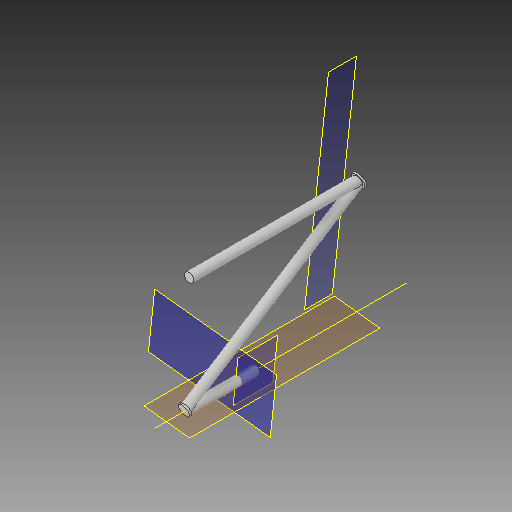
# Autodesk Inventor part: cellSTORM_lightpath
Saved by Autodesk Inventor 2019 (Build 230136000, 136)
## iProperties
Created: 2020-04-25
Part Number: cellSTORM_lightpath
Material: Generic
Document SubType Name: Modeling
Designer: diederichbenedict
Density: 1 g/cm^3
Appearance: Default
Author: diederichbenedict
Autodesk Inventor part; units mm, degrees
ref_plane "YZ Plane" through (0, 0, 0) normal (1, 0, 0) x (0, 1, 0)
ref_plane "XZ Plane" through (0, 0, 0) normal (0, 1, 0) x (-1, 0, 0)
ref_plane "XY Plane" through (0, 0, 0) normal (0, 0, 1) x (1, 0, 0)
ref_plane "Work Plane1" through (-18.0552, 1.9841, 10) normal (0, 0, -1) x (-0.9940164, 0.109231, 0)
ref_plane "Work Plane4" through (0, 0, 10) normal (-0.9940164, 0.109231, 0) x (-0.109231, -0.9940164, 0)
ref_plane "Work Plane3" through (-40.2485, 19.0101, 10) normal (-0.9940164, 0.109231, 0) x (-0.109231, -0.9940164, 0)
sketch "Sketch1" plane through (0, 0, 10) normal (-0.9940164, 0.109231, 0) x (-0.109231, -0.9940164, 0)
  line L0 (0, -10) -> (0, 30)
  line L1 (0, 30) -> (-70.8011, -60.6212)
  line L2 (-70.8011, -60.6212) -> (-70.8011, 34.3788)
  line L3 (-7.1094, 32.5876) -> (7.1094, 27.4124)
  line L4 (-78.8593, -57.6883) -> (-62.7428, -63.5542)
  dimension "d0" = 40
  dimension "d1" = 115
  dimension "d2" = 38
  dimension "d3" = 95
  dimension "d4" = 38
  dimension "d6" = 70
  constraints: 10 end point, 2 midpoint, 2 parallel, 1 vertical
  measures "d0" distance of L0.end L0.start
  measures "d1" distance of L0.end L1.end
  measures "d2" angle of L1 L0
  measures "d3" distance of L1.end L2.end
  measures "d4" angle of L1 L2
  measures "d6" angle of L3 L0
ref_plane "Work Plane7" through (-18.0552, 1.9841, 10) normal (0, 0, -1) x (-0.9940164, 0.109231, 0)
sketch "Sketch3" plane through (-18.0552, 1.9841, 10) normal (0, 0, -1) x (-0.9940164, 0.109231, 0)
  circle A0 centre (-18.1638, 0) radius 11.5 projected
  circle A1 centre (-18.1638, 0) radius 2.5
  point P0 (-18.1638, 0)
  dimension "d7" = 5
  constraints: 1 centre point, 1 coincident
  measures "d7" diameter of A1
sweep "Sweep1" add profiles "Sketch3" path "Sketch1" path curves L0 L1 L2 contours A1
ref_plane "Work Plane8" through (-22.055, 95.458, -62.5) normal (-0.9940164, 0.109231, 0) x (-0.109231, -0.9940164, 0)
sketch "Sketch4" plane through (-22.055, 95.458, -62.5) normal (-0.9940164, 0.109231, 0) x (-0.109231, -0.9940164, 0)
  line L0 (24.1767, 106.8788) -> (19.1767, 106.8788) projected
  line L1 (21.6767, 11.8788) -> (21.6767, 11.8788) projected
  line L2 (21.6767, 11.8788) -> (21.6767, 11.8788) projected
  line L3 (21.6767, 11.8788) -> (21.6767, 11.8788) projected
  line L4 (21.6767, 11.8788) -> (21.6767, 11.8788) projected
  line L5 (92.4778, 102.5) -> (92.4778, 102.5) projected
  line L6 (92.4778, 102.5) -> (92.4778, 102.5) projected
  line L7 (92.4778, 102.5) -> (92.4778, 102.5) projected
  line L8 (92.4778, 102.5) -> (92.4778, 102.5) projected
  line L9 (94.9778, 62.5) -> (89.9778, 62.5) projected
  line L10 (56.4279, -3) -> (16.4279, -3) projected
  line L11 (19.1767, 4.6182) -> (19.1767, 106.8788) projected
  line L12 (24.1767, 19.1393) -> (24.1767, 106.8788) projected
  line L13 (94.9778, 109.7605) -> (24.1767, 19.1393) projected
  line L14 (89.9778, 95.2395) -> (19.1767, 4.6182) projected
  line L15 (89.9778, 62.5) -> (89.9778, 95.2395) projected
  line L16 (94.9778, 62.5) -> (94.9778, 109.7605) projected
  line L17 (13.4434, 15.2665) -> (34.8257, 8.319)
  line L18 (34.8257, 8.319) -> (18.33, -8.9486)
  line L19 (18.33, -8.9486) -> (4.7452, 8.0853)
  line L20 (4.7452, 8.0853) -> (11.8837, 17.2222)
  line L21 (13.4434, 15.2665) -> (11.8837, 17.2222)
  line L22 (82.2165, 105.1215) -> (102.9149, 98.3962)
  line L23 (102.9149, 98.3962) -> (106.0468, 108.0351)
  line L24 (106.0468, 108.0351) -> (93.0792, 112.2485)
  line L25 (93.0792, 112.2485) -> (82.2165, 105.1215)
  point P0 (92.4778, 62.5)
  dimension "d10" = 70
  dimension "d11" = 7
  dimension "d12" = 7
  constraints: 18 end point, 2 parallel, 1 perpendicular, 1 point on line
  measures "d10" angle of L17 L14
  measures "d11" distance from line of L17 L12.start
  measures "d12" distance from line of L22 L15.end
extrude "Extrusion1" cut sketch "Sketch4" against normal through all contours L17 L14 L11 | L11 L14 L17 L18 L19 L20 L21 | L22 L25 L24 L23 L16 L13 | L13 L16 L22
sketch "Sketch5" plane through (7.7337, 70.3774, -49.9086) normal (0.0337542, 0.307168, -0.9510565) x (-0.9940164, 0.109231, 0)
  ellipse E0 centre (0, -0.4669) end of major axis (0, -3.1273) minor radius 2.5 (-2.4902, -0.232) -> (2.4902, -0.232) ccw projected
  ellipse E1 centre (0, 0) end of major axis (0, 2.6287) minor radius 2.5 (2.4902, -0.232) -> (-2.4902, -0.232) ccw projected
  line L0 (-2.4902, -0.1127) -> (2.4902, -0.1127) projected
  circle A0 centre (0, -0.1127) radius 3.7871
  point P0 (0, -51.9132)
  constraints: 1 centre point, 4 other
extrude "Extrusion2" add sketch "Sketch5" against normal blind 1 contours E1 E0 | A0
sketch "Sketch6" plane through (0.0485, 0.4414, 39.4317) normal (-0.0337542, -0.307168, 0.9510565) x (0.9940164, -0.109231, 0)
  ellipse E0 centre (0, 0) end of major axis (0, -2.6604) minor radius 2.5 (2.4902, -0.2348) -> (-2.4902, -0.2348) ccw projected
  ellipse E1 centre (0, -0.4669) end of major axis (0, 2.1618) minor radius 2.5 (-2.4902, -0.2348) -> (2.4902, -0.2348) ccw projected
  line L0 (-2.4902, -0.1127) -> (2.4902, -0.1127) projected
  circle A0 centre (0, -0.1127) radius 3.2394
  point P0 (0, -12.6073)
  constraints: 1 centre point, 4 other
extrude "Extrusion3" add sketch "Sketch6" against normal blind 1 contours E1 E0 | A0
ref_plane "Arbeitsebene10" through (0, 0, 0) normal (0.109231, 0.9940164, 0) x (0, 0, -1)
ref_plane "Arbeitsebene9" through (28.1562, 85.4859, 52.7288) normal (0.109231, 0.9940164, 0) x (0, 0, -1)
ref_plane "Work Plane2" through (-1.6385, -14.9102, 10) normal (0, 0, 1) x (0.9940164, -0.109231, 0)
body "Solid1"
